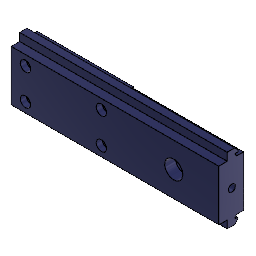
1-Belt_stepper_mount_Pt2_V3 v2 (Autodesk Fusion 360 design; units mm, degrees)
Autodesk Fusion 360 part; units mm, degrees
mesh "Mesh1" [no effect]
sketch "Sketch1" plane through (0, 0, 0) normal (1, 0, 0) x (0, 1, 0)
  line L0 (4.175, 6.1) -> (-4.2, 6.1)
  line L1 (4.175, 6.1) -> (9.6, 6.1)
  line L2 (-4.2, 6.1) -> (-10.775, 6.1)
  line L3 (-10.775, 6.1) -> (9.6, 6.1)
  line L4 (9.6, 6.1) -> (9.6, 45.6)
  line L5 (9.6, 45.6) -> (-10.775, 45.6)
  line L6 (-10.775, 45.6) -> (-10.775, 6.1)
  line L7 (-4.2, 45.6) -> (4.175, 45.6)
  line L8 (4.175, 45.6) -> (4.175, 51.7)
  line L9 (4.175, 51.7) -> (-4.2, 51.7)
  line L10 (-4.2, 51.7) -> (-4.2, 45.6)
  line L11 (1.625, 51.7) -> (4.175, 49.15)
  line L12 (1.625, 51.7) -> (5.4706, 51.7) construction
  line L13 (4.175, 49.15) -> (4.175, 47.85)
  line L14 (4.175, 47.85) -> (2.075, 47.85)
  line L15 (2.075, 47.85) -> (2.075, 47.2)
  line L16 (2.075, 47.2) -> (3.1141, 45.6)
  line L17 (-10.775, 25.85) -> (9.6, 25.85)
  line L18 (4.175, 0) -> (-4.2, 0)
  line L19 (2.075, 4.5) -> (3.1141, 6.1)
  line L20 (4.175, 3.85) -> (2.075, 3.85)
  line L21 (2.075, 3.85) -> (2.075, 4.5)
  line L22 (4.175, 2.55) -> (4.175, 3.85)
  line L23 (1.625, 0) -> (5.4706, 0) construction
  line L24 (4.175, 6.1) -> (4.175, 0)
  line L25 (1.625, 0) -> (4.175, 2.55)
  line L26 (-4.2, 0) -> (-4.2, 6.1)
  circle A0 centre (-0.5875, 25.85) radius 2.7
  dimension "d3" = 6.575
  dimension "d4" = 5.425
  dimension "d5" = 39.5
  dimension "d6" = 8.375
  dimension "d7" = 6.1
  dimension "d9" = 45
  dimension "d11" = 1.3
  dimension "d12" = 2.1
  dimension "d13" = 147
  dimension "d14" = 0.65
  dimension "d16" = 1.6
  dimension "d17" = 3.55
  dimension "d18" = 5.4
  constraint horizontal L0
  constraint horizontal L3
  constraint vertical L4
  constraint horizontal L5
  constraint vertical L6
  constraint horizontal L7
  constraint vertical L8
  constraint horizontal L9
  constraint vertical L10
  constraint coincident L5 L7.start
  constraint coincident L8 L11.end
  constraint parallel L8 L13
  constraint perpendicular L8 L14
  constraint perpendicular L14 L15
  constraint coincident L5 L16.end
  constraint midpoint L6 L17.start
  constraint midpoint L4 L17.end
  constraint perpendicular L4 L17
  constraint symmetric L7.start L17 L0.end
  constraint symmetric L7.end L17 L0.start
  constraint symmetric L8.end L17 L18.start
  constraint symmetric L9.end L17 L18.end
  constraint symmetric L11.start L17 L23.start
  constraint symmetric L12.end L17 L23.end
  constraint symmetric L11.end L17 L22.start
  constraint symmetric L13.end L17 L20.start
  constraint symmetric L14.end L17 L20.end
  constraint symmetric L15.end L17 L19.start
  constraint symmetric L16.end L17 L19.end
  constraint midpoint L17 A0.centre
  measures "d3" distance of L0.end L2.end
  measures "d4" distance of L0.start L1.end
  measures "d5" distance of L2.end L5.end
  measures "d6" distance of L7.start L7.end
  measures "d7" distance of L7.start L9.end
  measures "d9" angle of L11 L12
  measures "d11" distance of L11.end L13.end
  measures "d12" distance of L13.end L14.end
  measures "d13" angle of L15 L16
  measures "d14" distance of L14.end L15.end
  measures "d16" vertical distance of L15.end L16.end
  measures "d17" distance of L7.end L11.end
  measures "d18" diameter of A0
extrude "Extrude1" add sketch "Sketch1" against normal blind 161.5 contours L0 L1 L2 L3 L4 L6 L17 A0 | L0 L3 L18 L19 L20 L21 L22 L24 L25 L26 | L4 L5 L6 L7 L17 A0 | L17 A0 | L17 A0 | L5 L7 L8 L9 L10 L11 L13 L14 L15 L16
sketch "Sketch3" plane through (0, 9.6, 0) normal (0, 1, 0) x (1, 0, 0)
  circle A0 centre (-35.02, -25.8699) radius 17.75
  circle A1 centre (-35.02, -25.8699) radius 7
  line L0 (0, -6.1) -> (0, -45.6)
  line L1 (-10.225, -21.6) -> (-10.225, -30.1)
  line L2 (-10.225, -30.1) -> (-5.725, -30.1)
  line L3 (-5.725, -30.1) -> (-5.725, -21.6)
  line L4 (-5.725, -21.6) -> (-10.225, -21.6)
  line L5 (0, -25.85) -> (-162.2125, -25.85)
  circle A2 centre (-91.25, -37.85) radius 1.75
  line L6 (-91.25, -37.85) -> (-91.25, -25.85)
  line L7 (-91.25, -25.85) -> (-150.25, -25.85) construction
  line L8 (-150.25, -25.85) -> (-150.25, -37.85)
  circle A3 centre (-150.25, -37.85) radius 1.75
  circle A4 centre (-91.25, -13.85) radius 1.75
  circle A5 centre (-150.25, -13.85) radius 1.75
  circle A6 centre (-91.25, -37.85) radius 2.5
  circle A7 centre (-91.25, -37.85) radius 4
  circle A8 centre (-150.25, -37.85) radius 2.5
  circle A9 centre (-150.25, -37.85) radius 4
  circle A10 centre (-150.25, -13.85) radius 4
  circle A11 centre (-150.25, -13.85) radius 2.5
  circle A12 centre (-91.25, -13.85) radius 4
  circle A13 centre (-91.25, -13.85) radius 2.5
  line L9 (0, -45.6) -> (0, -6.1)
  line L10 (0, -6.1) -> (-161.5, -6.1)
  line L11 (-161.5, -6.1) -> (-161.5, -45.6)
  line L12 (-161.5, -45.6) -> (0, -45.6)
  line L13 (-10.225, -25.85) -> (-17.27, -25.85) construction
  line L14 (-86.445, -45.6) -> (-86.445, -6.1)
  line L15 (-52.77, -25.85) -> (-86.445, -25.85) construction
  point P0 (0, -25.85)
  dimension "d21" = 35.5
  dimension "d24" = 4.5
  dimension "d25" = 8.5
  dimension "d26" = 5.725
  dimension "d29" = 3.5
  dimension "d30" = 12
  dimension "d31" = 3.5
  dimension "d32" = 59
  dimension "d33" = 91.25
  dimension "d34" = 5
  dimension "d35" = 8
  dimension "d36" = 5
  dimension "d37" = 8
  dimension "d53" = 7.045
  dimension "d57" = 33.675
  constraint concentric A0 A1
  constraint horizontal L2
  constraint vertical L3
  constraint horizontal L4
  constraint coincident P0 L5.start
  constraint perpendicular L0 L5
  constraint coincident A2.centre L6.start
  constraint coincident L5 L6.end
  constraint perpendicular L5 L6
  constraint coincident L5 L7.end
  constraint perpendicular L5 L8
  constraint coincident L8.end A3.centre
  constraint symmetric L5 A2 A4
  constraint symmetric L5 A3 A5
  constraint concentric A2 A6
  constraint concentric A6 A7
  constraint symmetric L5 A6 A13
  constraint symmetric L5 A7 A12
  constraint symmetric L5 A8 A11
  constraint symmetric L5 A9 A10
  constraint midpoint L1 L13.start
  constraint coincident A0 L13.end
  constraint coincident L5 L13.end
  constraint perpendicular L1 L13
  constraint coincident L10 L14.end
  constraint perpendicular L10 L14
  constraint coincident A0 L15.start
  constraint coincident L5 L15.start
  constraint midpoint L14 L15.end
  constraint perpendicular L14 L15
  measures "d21" diameter of A0
  measures "d24" distance of L3.end L1.start
  measures "d25" distance of L1.start L1.end
  measures "d26" distance of L0 L3
  measures "d29" diameter of A2
  measures "d30" distance of L5 A2.centre
  measures "d31" diameter of A3
  measures "d32" distance of L6 L8
  measures "d33" distance of L0 L6
  measures "d34" diameter of A6
  measures "d35" diameter of A7
  measures "d36" diameter of A8
  measures "d37" diameter of A9
  measures "d53" distance of L13.start L13.end
  measures "d57" distance of L15.start L15.end
extrude "Extrude2" cut sketch "Sketch3" against normal blind 40 contours A1 L5 | A1 L5 | A2 | A3 | A4 | A5
extrude "Extrude4" cut sketch "Sketch3" against normal blind 12 contours A0 A1 L5 | A0 A1 L5
extrude "Extrude5" cut sketch "Sketch3" against normal blind 11 from surface at -11 contours A2 | A3 | A4 | A5 | A6 | A8 | A11 | A13
extrude "Extrude6" cut sketch "Sketch3" against normal blind 14 from surface at -15.8 contours A2 | A3 | A4 | A5 | A6 | A7 | A8 | A9 | A10 | A11 | A12 | A13
extrude "Extrude7" cut sketch "Sketch3" against normal blind 14.5 contours L1 L2 L3 L5 | L1 L3 L4 L5
extrude "Extrude8" cut sketch "Sketch3" against normal blind 1 contours A0 L0 L1 L2 L3 L5 L9 L12 L14 | A0 L0 L1 L3 L4 L5 L9 L10 L14
extrude "Extrude9" cut sketch "Sketch1" against normal blind 15.7 contours L17 A0 | L17 A0
sketch "Sketch4" plane through (0, 0, 0) normal (1, 0, 0) x (0, 1, 0)
  circle A0 centre (-0.5875, 25.85) radius 2.7
  line L0 (8.6, 6.1) -> (8.6, 45.6)
  line L1 (8.6, 45.6) -> (3.1141, 45.6)
  line L2 (3.1141, 45.6) -> (2.075, 47.2)
  line L3 (2.075, 47.2) -> (2.075, 47.85)
  line L4 (2.075, 47.85) -> (4.175, 47.85)
  line L5 (4.175, 47.85) -> (4.175, 49.15)
  line L6 (4.175, 49.15) -> (1.625, 51.7)
  line L7 (1.625, 51.7) -> (-4.2, 51.7)
  line L8 (-4.2, 51.7) -> (-4.2, 45.6)
  line L9 (-4.2, 45.6) -> (-10.775, 45.6)
  line L10 (-10.775, 45.6) -> (-10.775, 6.1)
  line L11 (-10.775, 6.1) -> (-4.2, 6.1)
  line L12 (-4.2, 6.1) -> (-4.2, 0)
  line L13 (-4.2, 0) -> (1.625, 0)
  line L14 (1.625, 0) -> (4.175, 2.55)
  line L15 (4.175, 2.55) -> (4.175, 3.85)
  line L16 (4.175, 3.85) -> (2.075, 3.85)
  line L17 (2.075, 3.85) -> (2.075, 4.5)
  line L18 (2.075, 4.5) -> (3.1141, 6.1)
  line L19 (3.1141, 6.1) -> (8.6, 6.1)
  circle A1 centre (-0.5875, 25.85) radius 2.75
  dimension "d62" = 5.5
  constraint concentric A0 A1
  measures "d62" diameter of A1
extrude "Extrude10" cut sketch "Sketch4" against normal blind 15.7 contours A1
equation "d25 = ( 4.25 * 2 ) * 1 mm"
